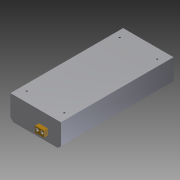
# Autodesk Inventor part: inverter
Saved by Autodesk Inventor 2012 (Build 160160000, 160)
## iProperties
Created: 2012-05-12
Part Number: inverter
Material: Default
Document SubType Name: Modeling
Designer: esv
Density: 1 g/cm^3
Author: esv
Autodesk Inventor part; units mm, degrees
ref_plane "YZ Plane" through (0, 0, 0) normal (1, 0, 0) x (0, 1, 0)
ref_plane "XZ Plane" through (0, 0, 0) normal (0, 1, 0) x (-1, 0, 0)
ref_plane "XY Plane" through (0, 0, 0) normal (0, 0, 1) x (1, 0, 0)
sketch "Sketch1" plane through (0, 0, 0) normal (0, 0, 1) x (1, 0, 0)
  line L0 (9.525, 0) -> (152.4, 0)
  line L1 (161.925, 9.525) -> (161.925, 76.2)
  line L2 (161.925, 76.2) -> (0, 76.2)
  line L3 (0, 76.2) -> (0, 9.525)
  line L4 (9.525, 0) -> (0, 9.525)
  line L5 (161.925, 9.525) -> (152.4, 0)
  point P0 (0, 0)
  point P1 (161.925, 0)
  dimension "d0" = 161.925
  dimension "d1" = 76.2
  dimension "d2" = 9.525
  dimension "d3" = 9.525
  dimension "d4" = 9.525
  dimension "d5" = 9.525
  constraints: 12 end point, 4 point on line, 2 parallel, 1 horizontal, 1 perpendicular
  measures "d0" distance of point (0, 0) point (161.925, 0)
  measures "d1" distance of point (161.925, 0) L1.end
  measures "d2" distance of L0.start point (0, 0)
  measures "d3" distance of L3.end point (0, 0)
  measures "d4" distance of L1.start point (161.925, 0)
  measures "d5" distance of L0.end point (161.925, 0)
extrude "Main Body" add sketch "Sketch1" along normal blind 361.95
sketch "Sketch2" plane through (0, 0, 361.95) normal (0, 0, 1) x (1, 0, 0)
  line L0 (161.925, 76.2) -> (161.925, 9.525) projected
  line L1 (152.4, 0) -> (9.525, 0) projected
  line L2 (92.075, 38.1) -> (120.65, 38.1)
  line L3 (120.65, 38.1) -> (120.65, 19.05)
  line L4 (120.65, 19.05) -> (92.075, 19.05)
  line L5 (92.075, 19.05) -> (92.075, 38.1)
  point P0 (0, 0)
  dimension "d8" = 41.275
  dimension "d9" = 19.05
  dimension "d10" = 28.575
  dimension "d11" = 19.05
  constraints: 8 end point, 2 parallel, 1 horizontal, 1 perpendicular
  measures "d8" distance between parallel lines of L0 L3
  measures "d9" distance between parallel lines of L1 L4
  measures "d10" distance of L3.end L4.end
  measures "d11" distance of L2.end L3.end
extrude "Terminal Block" add sketch "Sketch2" along normal blind 12.7
sketch "Sketch3" plane through (0, 0, 374.65) normal (0, 0, 1) x (1, 0, 0)
  line L0 (92.075, 38.1) -> (120.65, 38.1) projected
  line L1 (98.425, 30.1625) -> (114.3, 30.1625)
  point P0 (0, 0)
  point P1 (106.3625, 30.1625)
  point P2 (106.3625, 38.1)
  dimension "d14" = 15.875
  dimension "d15" = 7.9375
  constraints: 2 end point, 2 midpoint, 1 horizontal, 1 vertical alignment
  measures "d14" distance of L1.end L1.start
  measures "d15" distance between parallel lines of L0 L1
hole "Terminal Holes" at (98.425, 30.1625, 374.65) at (114.3, 30.1625, 374.65) direction (0, 0, -1) diameter 9.525 depth 12.7 tip angle 118
sketch "Sketch4" plane through (0, 76.2, 0) normal (0, 1, 0) x (1, 0, 0)
  line L0 (0, 0) -> (161.925, 0) projected
  line L1 (0, 0) -> (0, -361.95) projected
  line L2 (20.6375, -31.75) -> (141.2875, -31.75)
  line L3 (141.2875, -31.75) -> (141.2875, -330.2)
  line L4 (141.2875, -330.2) -> (20.6375, -330.2)
  line L5 (20.6375, -330.2) -> (20.6375, -31.75)
  point P0 (20.6375, -180.975)
  point P1 (0, -180.975)
  point P2 (80.9625, 0)
  point P3 (80.9625, -31.75)
  dimension "d23" = 120.65
  dimension "d24" = 298.45
  constraints: 8 end point, 4 coincident, 4 midpoint, 2 parallel, 1 horizontal, 1 horizontal alignment, 1 perpendicular, 1 vertical alignment
  measures "d23" distance of L2.start L2.end
  measures "d24" distance of L4.end L2.start
hole "Hole2" at (20.6375, 76.2, 31.75) at (141.2875, 76.2, 31.75) at (141.2875, 76.2, 330.2) at (20.6375, 76.2, 330.2) direction (0, -1, 0) diameter 4.9784 depth 25.4 tip angle 118 thread size "1/4-20 UNC" class "2B" standard "ANSI Unified Screw Threads"
equation "\"d3\" = d2"
equation "\"d4\" = d2"
equation "\"d5\" = d4"
body "Solid1"
